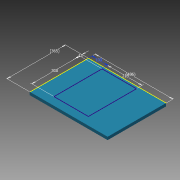
# Autodesk Inventor part: base
Saved by Autodesk Inventor 2013 SP2 (Build 170200200, 200)
## iProperties
Created: 2017-01-25
Part Number: base
Material: Generic
Document SubType Name: Modeling
Designer: Herman de Vries
Density: 1 g/cm^3
Mass: 3888 g
Surface Area: 4654.8 cm^2
Volume: 3888 cm^3
Author: Herman de Vries
Autodesk Inventor part; units mm, degrees
ref_plane "YZ Plane" through (0, 0, 0) normal (1, 0, 0) x (0, 1, 0)
ref_plane "XZ Plane" through (0, 0, 0) normal (0, 1, 0) x (-1, 0, 0)
ref_plane "XY Plane" through (0, 0, 0) normal (0, 0, 1) x (1, 0, 0)
sketch "Sketch1" plane through (0, 0, 0) normal (0, 0, 1) x (1, 0, 0)
  line L0 (0, 0) -> (486, 0)
  line L1 (486, 0) -> (486, 365)
  line L2 (486, 365) -> (0, 365)
  line L3 (0, 365) -> (0, 0)
  dimension "d0" = 486
  dimension "d1" = 365
  constraints: 8 end point, 2 parallel, 1 horizontal, 1 perpendicular
  measures "d0" distance of L2.end L1.end
  measures "d1" distance of L1.end L0.end
extrude "Extrusion1" add sketch "Sketch1" along normal blind 18
sketch "Sketch2" plane through (0, 0, 18) normal (0, 0, 1) x (1, 0, 0)
  line L0 (100, 50) -> (315, 50)
  line L1 (315, 50) -> (315, 350)
  line L2 (315, 350) -> (100, 350)
  line L3 (100, 350) -> (100, 50)
  line L4 (486, 365) -> (0, 365) projected
  line L5 (0, 365) -> (0, 0) projected
  dimension "d4" = 300
  dimension "d6" = 215
  dimension "d7" = 15
  dimension "d8" = 100
  dimension "d9" = 486
  dimension "d10" = 365
  constraints: 8 end point, 2 parallel, 1 horizontal, 1 perpendicular
  measures "d4" distance of L2.end L0.start
  measures "d6" distance of L1.end L2.end
  measures "d7" distance from line of L2.end L4
  measures "d8" distance between parallel lines of L5 L3
  measures "d9" distance of L4.start L4.end
  measures "d10" distance of L4.end L5.end
body "Solid1"
